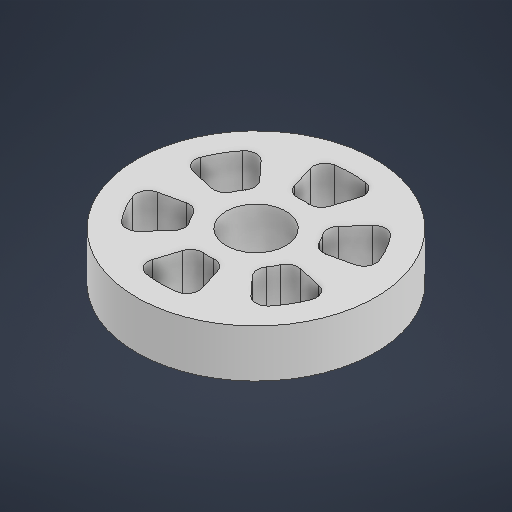
# Autodesk Inventor part: 2.5in flex
Saved by Autodesk Inventor 2025.2 (Build 292293000, 293)
## iProperties
Created: 2025-12-04
Part Number: 2.5in flex
Material: Generic
Document SubType Name: Modeling
Designer: cloudy
Density: 1 g/cm^3
Appearance: Default
Author: cloudy
Autodesk Inventor part; units mm, degrees
ref_plane "YZ Plane" through (0, 0, 0) normal (1, 0, 0) x (0, 1, 0)
ref_plane "XZ Plane" through (0, 0, 0) normal (0, 1, 0) x (-1, 0, 0)
ref_plane "XY Plane" through (0, 0, 0) normal (0, 0, 1) x (1, 0, 0)
sketch "Sketch1" plane through (0, 0, 0) normal (0, 1, 0) x (-1, 0, 0)
  circle A0 centre (0, 0) radius 31.75
  circle A1 centre (0, 0) radius 12.7
  circle A2 centre (0, 0) radius 25.4
  line L0 (24.7979, 5.4976) -> (12.399, 2.7488)
  line L1 (12.399, -2.7488) -> (24.7979, -5.4976)
  circle A3 centre (0, 0) radius 7.9375
  line L2 (0, 0) -> (7.9375, 0) construction
  line L3 (8.58, 9.3634) -> (17.16, 18.7268)
  line L4 (7.6379, 24.2244) -> (3.819, 12.1122)
  line L5 (-3.819, 12.1122) -> (-7.6379, 24.2244)
  line L6 (-17.16, 18.7268) -> (-8.58, 9.3634)
  line L7 (-12.399, 2.7488) -> (-24.7979, 5.4976)
  line L8 (-24.7979, -5.4976) -> (-12.399, -2.7488)
  line L9 (-8.58, -9.3634) -> (-17.16, -18.7268)
  line L10 (-7.6379, -24.2244) -> (-3.819, -12.1122)
  line L11 (3.819, -12.1122) -> (7.6379, -24.2244)
  line L12 (17.16, -18.7268) -> (8.58, -9.3634)
  dimension "d3" = 15.875
  dimension "d0" = 63.5
  dimension "d1" = 25.4
  dimension "d2" = 50.8
  dimension "d4" = 25
  dimension "d7" = 360
  constraints: 26 end point, 12 point on line, 6 coincident, 4 point on circle, 3 centre point, 1 horizontal, 1 horizontal alignment, 44 other
  measures "d0" diameter of A0
  measures "d1" diameter of A1
  measures "d2" diameter of A2
  measures "d4" angle of L1 L0
extrude "Extrusion1" add sketch "Sketch1" along normal blind 12.7 contours A0 | A1 | A1 L0 A2 L1 | A1 L4 A2 L3 | L12 A2 L11 A1 | A1 L6 A2 L5 | L10 A2 L9 A1 | A1 L8 A2 L7
fillet "Fillet1" radius 3.175 4 edges at (-3.819, 6.35, -12.1122) (3.819, 6.35, -12.1122) (7.6379, 6.35, -24.2244) (-7.6379, 6.35, -24.2244)
pattern_circular "Circular Pattern1" count 6 over 360 about axis through (0, 0, 0) along (0, 1, 0) of "Fillet1"
body "Solid1"
